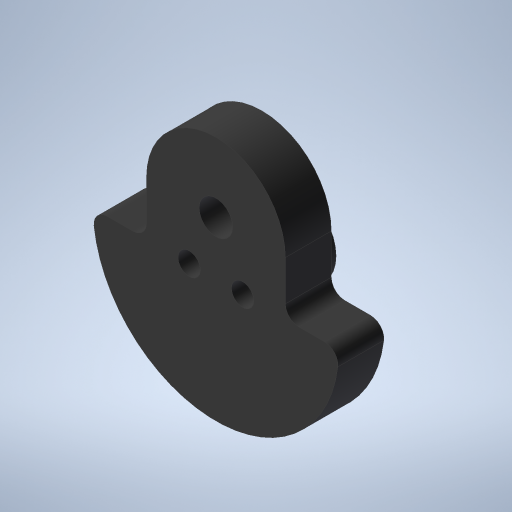
# Autodesk Inventor part: Crank on Crankshaft 2
Saved by Autodesk Inventor 2023 (Build 270158000, 158)
## iProperties
Created: 2022-10-29
Part Number: Crank on Crankshaft 2
Material: Generic
Document SubType Name: Modeling
Designer: tommy
Density: 1 g/cm^3
Appearance: Default
Author: tommy
## iProperties of the stored document Crank on Crankshaft_3DPrint.ipt
Created: 2022-10-29
Part Number: Crank on Crankshaft_3DPrint
Material: Generic
Document SubType Name: Modeling
Designer: tommy
Density: 1 g/cm^3
Appearance: Default
Author: tommy
Autodesk Inventor part; units mm, degrees
ref_plane "YZ Plane" through (0, 0, 0) normal (1, 0, 0) x (0, 1, 0)
ref_plane "XZ Plane" through (0, 0, 0) normal (0, 1, 0) x (-1, 0, 0)
ref_plane "XY Plane" through (0, 0, 0) normal (0, 0, 1) x (1, 0, 0)
sketch "Sketch1" plane through (0, 0, 0) normal (0, 0, 1) x (1, 0, 0)
  circle A0 centre (0, 12.7) radius 3.9878
  circle A1 centre (-6.35, 0) radius 1.5875
  circle A2 centre (6.35, 0) radius 1.5875
  circle A3 centre (0, 0) radius 9.525
  arc A4 (-28.992, -3.5622) -> (28.992, -3.5622) centre (0, 0) ccw
  line L0 (-16.51, 12.7) -> (-16.51, 3.175)
  line L1 (16.51, 12.7) -> (16.51, 3.175)
  line L2 (19.685, 0) -> (25.8407, 0)
  line L3 (-19.685, 0) -> (-25.8407, 0)
  arc A5 (16.51, 12.7) -> (-16.51, 12.7) centre (0, 12.7) ccw
  arc A6 (-25.8407, 0) -> (-28.992, -3.5622) centre (-25.8407, -3.175) ccw
  arc A7 (-19.685, 0) -> (-16.51, 3.175) centre (-19.685, 3.175) ccw
  arc A8 (16.51, 3.175) -> (19.685, 0) centre (19.685, 3.175) ccw
  arc A9 (28.992, -3.5622) -> (25.8407, 0) centre (25.8407, -3.175) ccw
  circle A10 centre (6.35, 0) radius 2.667
  circle A11 centre (-6.35, 0) radius 2.667
  circle A12 centre (0, 12.7) radius 9.398
  point P0 (-9.525, 0)
  point P1 (9.525, 0)
  point P2 (-16.51, -24.0966)
  point P3 (16.51, -24.0966)
  point P4 (-29.21, 0)
  point P5 (29.21, 0)
  point P6 (-2.077, 9.2958)
  point P7 (2.077, 9.2958)
  point P8 (7.0137, 6.4446)
  point P9 (-7.0137, 6.4446)
  dimension "d20" = 7.9756
  dimension "d44" = 3.175
  dimension "d51" = 5.334
  dimension "d52" = 5.334
  dimension "d57" = 18.796
  constraints: 16 point on circle, 12 centre point, 8 end point, 8 tangent, 4 coincident, 4 point on line, 3 equal radius, 2 horizontal, 2 vertical, 3 other
  measures "d20" diameter of A0
  measures "d44" radius of A6
  measures "d51" diameter of A10
  measures "d52" diameter of A11
  measures "d57" diameter of A12
extrude "Extrusion9" add sketch "Sketch1" along normal blind 19.05 contours A0 A3 | A0 A3 A12 | A3 A0 | A0 A3 A12 | A12 A3 | A1 | A2 | A6 L3 A7 L0 A5 L1 A8 L2 A9 A4 | A10 | A11
extrude "Extrusion10" cut sketch "Sketch1" along normal blind 8.128 contours A0 A3 | A0 A3 A12 | A3 A0 | A0 A3 A12 | A6 L3 A7 L0 A5 L1 A8 L2 A9 A4
extrude "Extrusion11" cut sketch "Sketch1" along normal blind 38.1 contours A0 A3 | A3 A0
extrude "Extrusion12" cut sketch "Sketch1" along normal blind 38.1 contours A1 | A2 | A10 | A11
extrude "Extrusion13" add sketch "Sketch1" along normal blind 9.525 contours A10 | A11
fillet "Fillet2" radius 3.175 1 edges at (0, -9.525, 8.128)
body "Solid4"
